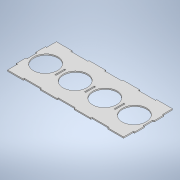
# Autodesk Inventor part: base
Saved by Autodesk Inventor 2020 (Build 240168000, 168)
## iProperties
Created: 2020-02-22
Part Number: base
Material: Generic
Document SubType Name: Modeling
Designer: udvarhelyi
Density: 1 g/cm^3
Appearance: Default
Author: udvarhelyi
Autodesk Inventor part; units mm, degrees
ref_plane "YZ Plane" through (0, 0, 0) normal (1, 0, 0) x (0, 1, 0)
ref_plane "XZ Plane" through (0, 0, 0) normal (0, 1, 0) x (-1, 0, 0)
ref_plane "XY Plane" through (0, 0, 0) normal (0, 0, 1) x (1, 0, 0)
sketch "Sketch1" plane through (0, 0, 0) normal (0, 1, 0) x (-1, 0, 0)
  line L0 (107.1429, 58.8466) -> (107.1429, 61.8466)
  line L1 (64.2857, 61.8466) -> (64.2857, 58.8466)
  line L2 (21.4286, 58.8466) -> (21.4286, 61.8466)
  line L3 (-21.4286, 61.8466) -> (-21.4286, 58.8466)
  line L4 (-64.2857, 61.8466) -> (-64.2857, 58.8466)
  line L5 (-107.1429, 58.8466) -> (-107.1429, 61.8466)
  line L6 (107.1429, -58.8466) -> (107.1429, -61.8466)
  line L7 (64.2857, -58.8466) -> (64.2857, -61.8466)
  line L8 (21.4286, -58.8466) -> (21.4286, -61.8466)
  line L9 (-21.4286, -58.8466) -> (-21.4286, -61.8466)
  line L10 (-64.2857, -58.8466) -> (-64.2857, -61.8466)
  line L11 (-107.1429, -58.8466) -> (-107.1429, -61.8466)
  line L12 (107.1429, 61.8466) -> (147, 61.8466)
  line L13 (107.1429, 58.8466) -> (64.2857, 58.8466)
  line L14 (147, -61.8466) -> (107.1429, -61.8466)
  line L15 (64.2857, -61.8466) -> (21.4286, -61.8466)
  line L16 (-21.4286, -61.8466) -> (-64.2857, -61.8466)
  line L17 (-107.1429, -61.8466) -> (-147, -61.8466)
  line L18 (64.2857, -58.8466) -> (107.1429, -58.8466)
  line L19 (-107.1429, -58.8466) -> (-64.2857, -58.8466)
  line L20 (-21.4286, -58.8466) -> (21.4286, -58.8466)
  line L21 (21.4286, 61.8466) -> (64.2857, 61.8466)
  line L22 (21.4286, 58.8466) -> (-21.4286, 58.8466)
  line L23 (-64.2857, 58.8466) -> (-107.1429, 58.8466)
  line L24 (-147, 61.8466) -> (-107.1429, 61.8466)
  line L25 (-64.2857, 61.8466) -> (-21.4286, 61.8466)
  line L26 (147, 37.108) -> (150, 37.108)
  line L27 (150, 12.3693) -> (147, 12.3693)
  line L28 (147, -12.3693) -> (150, -12.3693)
  line L29 (150, -37.108) -> (147, -37.108)
  line L30 (147, -37.108) -> (147, -61.8466)
  line L31 (150, 37.108) -> (150, 12.3693)
  line L32 (150, -12.3693) -> (150, -37.108)
  line L33 (147, 61.8466) -> (147, 37.108)
  line L34 (147, 12.3693) -> (147, -12.3693)
  line L35 (-147, -37.108) -> (-150, -37.108)
  line L36 (-150, -12.3693) -> (-147, -12.3693)
  line L37 (-147, 12.3693) -> (-150, 12.3693)
  line L38 (-150, 37.108) -> (-147, 37.108)
  line L39 (-150, 37.108) -> (-150, 12.3693)
  line L40 (-150, -12.3693) -> (-150, -37.108)
  line L41 (-147, 37.108) -> (-147, 61.8466)
  line L42 (-147, -61.8466) -> (-147, -37.108)
  line L43 (-147, -12.3693) -> (-147, 12.3693)
  point P0 (0, 0)
  dimension "d23" = 123.6932
  dimension "d35" = 3
  dimension "d36" = 61.8466
  dimension "d37" = 3
  dimension "d41" = 24.7386
  dimension "d42" = 49.4773
  dimension "d43" = 74.2159
  dimension "d44" = 98.9545
  dimension "d45" = 3
  dimension "d46" = 42.8571
  dimension "d47" = 128.5714
  dimension "d48" = 171.4286
  dimension "d49" = 214.2857
  dimension "d50" = 85.7143
  dimension "d51" = 257.1429
  dimension "d52" = 300
  dimension "d53" = 3
  dimension "d54" = 150
  constraints: 88 end point, 62 perpendicular, 27 parallel, 26 collinear, 4 horizontal, 4 vertical
  measures "d23" distance between parallel lines of L12 L14
  measures "d35" distance of L11.start L11.end
  measures "d36" distance from line of L16 point (0, 0)
  measures "d37" distance of L0.start L0.end
  measures "d41" distance from line of L26.start L12
  measures "d42" distance from line of L12 L27.end
  measures "d43" distance between parallel lines of L12 L28
  measures "d44" distance from line of L12 L29.start
  measures "d45" distance of L26.start L26.end
  measures "d46" distance from line of L0.end L31
  measures "d47" distance from line of L31 L2.end
  measures "d48" distance from line of L31 L3.start
  measures "d49" distance from line of L31 L4.start
  measures "d50" distance from line of L31 L1.start
  measures "d51" distance from line of L31 L5.end
  measures "d52" distance between parallel lines of L39 L31
  measures "d53" distance of L38.start L38.end
  measures "d54" distance from line of point (0, 0) L32
extrude "Extrusion1" add sketch "Sketch1" along normal blind 3
sketch "Sketch2" plane through (0, 3, 0) normal (0, 1, 0) x (1, 0, 0)
  ellipse E0 centre (-112.5, 0) end of major axis (-112.5, 30.9233) minor radius 30
  point P0 (0, 0)
  point P1 (-82.5, 0)
  point P2 (-112.5, -30.9233)
  dimension "d55" = 112.5
  dimension "d56" = 30
  dimension "d57" = 30.9233
  constraints: 4 other
  measures "d55" distance of point (0, 0) point (-112.5, 0)
  measures "d56" distance of point (-112.5, 0) point (-82.5, 0)
  measures "d57" distance of point (-112.5, 0) point (-112.5, -30.923)
extrude "Extrusion2" cut sketch "Sketch2" against normal through all
pattern_linear "Rectangular Pattern1" count 4 spacing 75 along (1, 0, 0) of "Extrusion2"
sketch "Sketch3" plane through (0, 3, 0) normal (0, 1, 0) x (1, 0, 0)
  line L0 (-76.5, -12.3693) -> (-73.5, -12.3693)
  line L1 (-73.5, -12.3693) -> (-73.5, 12.3693)
  line L2 (-73.5, 12.3693) -> (-76.5, 12.3693)
  line L3 (-76.5, 12.3693) -> (-76.5, -12.3693)
  point P0 (0, 0)
  dimension "d92" = 24.7386
  dimension "d93" = 73.5
  dimension "d94" = 3
  dimension "d95" = 12.3693
  constraints: 8 end point, 2 parallel, 1 horizontal, 1 perpendicular
  measures "d92" distance of L2.end L0.start
  measures "d93" distance from line of point (0, 0) L1
  measures "d94" distance of L0.start L0.end
  measures "d95" distance from line of point (0, 0) L2
extrude "Extrusion3" cut sketch "Sketch3" against normal through all
pattern_linear "Rectangular Pattern2" count 3 spacing 75 along (1, 0, 0) of "Extrusion3"
equation "\"d23\" = dt"
equation "\"d35\" = tt"
equation "\"d36\" = 0.5 * dt"
equation "\"d37\" = tt"
equation "\"d41\" = 0.2 * dt - tol"
equation "\"d42\" = 0.4 * dt + tol"
equation "\"d43\" = 0.6 * dt - tol"
equation "\"d44\" = 0.8 * dt + tol"
equation "\"d45\" = tt"
equation "\"d46\" = 0.142857 * wt + tol"
equation "\"d47\" = 0.428571 * wt + tol"
equation "\"d48\" = 0.571429 * wt - tol"
equation "\"d49\" = 0.714286 * wt + tol"
equation "\"d50\" = 0.285714 * wt - tol"
equation "\"d51\" = 0.857143 * wt - tol"
equation "\"d52\" = wt"
equation "\"d53\" = tt"
equation "\"d54\" = 0.5 * wt"
equation "\"d31\" = tt"
equation "\"d56\" = 0.5 * glassDia"
equation "\"d92\" = 0.2 * dt + 2 * tol"
equation "\"d93\" = 0.25 * wt - 0.5 * tt"
equation "\"d94\" = tt"
equation "\"d95\" = 0.1 * dt + tol"
equation "\"d100\" = 0.25 * wt"
equation "\"d0\" = 0.5 * dt"
equation "\"d1\" = 0.5 * dt"
equation "\"d4\" = tt"
equation "\"wt\" = 300"
equation "\"tt\" = 3"
equation "\"tol\" = 0"
equation "\"tiroir\" = 1"
equation "\"d39\" = tt"
equation "\"d40\" = tt"
equation "\"nHoles\" = 4"
equation "\"shelfH\" = 35"
equation "\"dt\" = 123.693169"
equation "\"glassDia\" = 60"
body "Solid1"
